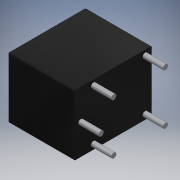
# Autodesk Inventor part: VAR-RELAY-12V10A-CHICO
Saved by Autodesk Inventor 2018.3 (Build 223284000, 284)
## iProperties
Created: 2021-05-31
Part Number: VAR-RELAY-12V10A-CHICO
Material: Genérico
Document SubType Name: Modeling
Designer: laguerre
Density: 8.47 g/cm^3
Appearance: Suave - Negro
Author: laguerre
Autodesk Inventor part; units mm, degrees
note: some values were not read from the file. Chosen so that the rebuilt part matches the saved one: direction of "Repujado1".
ref_plane "YZ Plane" through (0, 0, 0) normal (1, 0, 0) x (0, 1, 0)
ref_plane "XZ Plane" through (0, 0, 0) normal (0, 1, 0) x (-1, 0, 0)
ref_plane "XY Plane" through (0, 0, 0) normal (0, 0, 1) x (1, 0, 0)
sketch "Boceto39" plane through (0, 0, 0) normal (0, 0, 1) x (1, 0, 0)
  line L0 (-7.65, 6) -> (7.65, 6)
  line L1 (7.65, 6) -> (7.65, -6)
  line L2 (7.65, -6) -> (-7.65, -6)
  line L3 (-7.65, -6) -> (-7.65, 6)
  point P0 (0, 0)
  point P1 (0, 6)
  point P2 (-7.65, 0)
  dimension "d373" = 15.3
  dimension "d374" = 12
  constraints: 8 end point, 2 midpoint, 2 parallel, 1 horizontal, 1 horizontal alignment, 1 perpendicular, 1 vertical alignment
  measures "d373" distance of L0.start L0.end
  measures "d374" distance of L2.end L0.start
extrude "Extrusión13" add sketch "Boceto39" along normal blind 13.1
sketch "Boceto40" plane through (0, 0, 0) normal (0, 0, -1) x (-1, 0, 0)
  circle A0 centre (-6.35, 0) radius 0.5
  circle A1 centre (-3.85, 5) radius 0.5
  circle A2 centre (-3.85, -5) radius 0.5
  circle A3 centre (6.35, -5) radius 0.5
  circle A4 centre (6.35, 5) radius 0.5
  line L0 (-7.65, 6) -> (-7.65, -6) projected
  point P0 (0, 0)
  dimension "d377" = 2.5
  dimension "d378" = 10.2
  dimension "d379" = 10
  dimension "d380" = 5
  dimension "d381" = 1
  dimension "d382" = 1.3
  constraints: 5 centre point, 4 equal radius, 3 horizontal alignment, 2 vertical alignment
  measures "d377" horizontal distance of A2.centre A0.centre
  measures "d378" distance of A3.centre A2.centre
  measures "d379" distance of A1.centre A2.centre
  measures "d380" vertical distance of A1.centre A0.centre
  measures "d381" diameter of A1
  measures "d382" distance from line of A0.centre L0
extrude "Extrusión14" add sketch "Boceto40" along normal blind 4
fillet "Empalme44" radius 0.2 8 edges at (7.65, 6, 6.55) (7.65, -6, 6.55) (-7.65, 6, 6.55) (-7.65, -6, 6.55) (-7.65, 0, 13.1) (0, -6, 13.1) (7.65, 0, 13.1) (0, 6, 13.1)
sketch "Boceto41" plane through (0, 0, 13.1) normal (0, 0, 1) x (1, 0, 0)
  line L0 (5.3129, 0) -> (-7.1764, 0) construction
  line L1 (-7.1764, 0) -> (-7.1764, 5.3526) construction
  line L2 (-7.1764, 5.3526) -> (5.3129, 5.3526) construction
  line L3 (5.3129, 5.3526) -> (5.3129, 0) construction
  line L4 (4.6233, 1.0211) -> (5.24, 1.0211)
  line L5 (5.24, 1.0211) -> (5.24, 0.8793)
  spline S0 degree 2 poles (5.24, 0.8793) (5.1736, 0.8169) (5.0552, 0.701) (4.9985, 0.6386) knots 0 0 0 1 2 2 2
  spline S1 degree 2 poles (4.9985, 0.6386) (4.8843, 0.513) (4.8008, 0.3622) (4.8008, 0.282) knots 0 0 0 1 2 2 2
  spline S2 degree 2 poles (4.8008, 0.282) (4.8008, 0.2399) (4.8267, 0.1767) (4.8502, 0.1564) knots 0 0 0 1 2 2 2
  spline S3 degree 2 poles (4.8502, 0.1564) (4.8737, 0.1361) (4.9353, 0.1159) (4.9726, 0.1159) knots 0 0 0 1 2 2 2
  spline S4 degree 2 poles (4.9726, 0.1159) (5.0082, 0.1159) (5.0812, 0.1337) (5.1144, 0.1475) knots 0 0 0 1 2 2 2
  spline S5 degree 2 poles (5.1144, 0.1475) (5.1428, 0.1588) (5.1954, 0.1912) (5.2116, 0.2026) knots 0 0 0 1 2 2 2
  line L6 (5.2116, 0.2026) -> (5.2189, 0.2026)
  line L7 (5.2189, 0.2026) -> (5.2189, 0.06)
  spline S6 degree 2 poles (5.2189, 0.06) (5.1776, 0.0397) (5.0293, 0) (4.9629, 0) knots 0 0 0 1 2 2 2
  spline S7 degree 2 poles (4.9629, 0) (4.8227, 0) (4.6646, 0.1483) (4.6646, 0.2747) knots 0 0 0 1 2 2 2
  spline S8 degree 2 poles (4.6646, 0.2747) (4.6646, 0.3339) (4.6922, 0.4327) (4.7165, 0.4749) knots 0 0 0 1 2 2 2
  spline S9 degree 2 poles (4.7165, 0.4749) (4.7408, 0.5186) (4.8113, 0.6045) (4.8502, 0.6459) knots 0 0 0 1 2 2 2
  spline S10 degree 2 poles (4.8502, 0.6459) (4.9134, 0.7147) (5.0682, 0.8622) (5.1144, 0.9052) knots 0 0 0 1 2 2 2
  line L8 (5.1144, 0.9052) -> (4.6233, 0.9052)
  line L9 (4.6233, 0.9052) -> (4.6233, 1.0211)
  spline S11 degree 2 poles (3.8672, 0.5211) (3.8672, 0.7901) (4.0236, 1.0421) (4.1865, 1.0421) knots 0 0 0 1 2 2 2
  spline S12 degree 2 poles (4.1865, 1.0421) (4.3518, 1.0421) (4.5066, 0.7853) (4.5066, 0.5219) knots 0 0 0 1 2 2 2
  spline S13 degree 2 poles (4.5066, 0.5219) (4.5066, 0.2512) (4.3502, 0.0008) (4.1865, 0.0008) knots 0 0 0 1 2 2 2
  spline S14 degree 2 poles (4.1865, 0.0008) (4.022, 0.0008) (3.8672, 0.2601) (3.8672, 0.5211) knots 0 0 0 1 2 2 2
  spline S15 degree 2 poles (4.039, 0.8258) (4.0196, 0.7763) (4.0034, 0.624) (4.0034, 0.5211) knots 0 0 0 1 2 2 2
  spline S16 degree 2 poles (4.0034, 0.5211) (4.0034, 0.4182) (4.0196, 0.2666) (4.0398, 0.2156) knots 0 0 0 1 2 2 2
  spline S17 degree 2 poles (4.0398, 0.2156) (4.0601, 0.1645) (4.1306, 0.1118) (4.1865, 0.1118) knots 0 0 0 1 2 2 2
  spline S18 degree 2 poles (4.1865, 0.1118) (4.2424, 0.1118) (4.3146, 0.1645) (4.3356, 0.2172) knots 0 0 0 1 2 2 2
  spline S19 degree 2 poles (4.3356, 0.2172) (4.3559, 0.2682) (4.3705, 0.4238) (4.3705, 0.5219) knots 0 0 0 1 2 2 2
  spline S20 degree 2 poles (4.3705, 0.5219) (4.3705, 0.6272) (4.3575, 0.7682) (4.3364, 0.8233) knots 0 0 0 1 2 2 2
  spline S21 degree 2 poles (4.3364, 0.8233) (4.317, 0.8752) (4.2449, 0.9311) (4.1865, 0.9311) knots 0 0 0 1 2 2 2
  spline S22 degree 2 poles (4.1865, 0.9311) (4.1314, 0.9311) (4.0593, 0.8784) (4.039, 0.8258) knots 0 0 0 1 2 2 2
  line L10 (3.8186, 1.0211) -> (3.4815, 0.0211)
  line L11 (3.4815, 0.0211) -> (3.3178, 0.0211)
  line L12 (3.3178, 0.0211) -> (2.9807, 1.0211)
  line L13 (2.9807, 1.0211) -> (3.1209, 1.0211)
  line L14 (3.1209, 1.0211) -> (3.2116, 0.7415)
  line L15 (3.2116, 0.7415) -> (3.5933, 0.7415)
  line L16 (3.5933, 0.7415) -> (3.6841, 1.0211)
  line L17 (3.6841, 1.0211) -> (3.8186, 1.0211)
  line L18 (3.2481, 0.628) -> (3.4029, 0.1572)
  line L19 (3.4029, 0.1572) -> (3.5569, 0.628)
  line L20 (3.5569, 0.628) -> (3.2481, 0.628)
  line L21 (0.2003, 1.0211) -> (0.6881, 1.0211)
  line L22 (0.6881, 1.0211) -> (0.6881, 0.919)
  line L23 (0.6881, 0.919) -> (0.5066, 0.919)
  line L24 (0.5066, 0.919) -> (0.5066, 0.2488)
  line L25 (0.5066, 0.2488) -> (0.6881, 0.2488)
  line L26 (0.6881, 0.2488) -> (0.6881, 0.1572)
  spline S23 degree 2 poles (0.6881, 0.1572) (0.5852, 0.1572) (0.488, 0.0989) (0.4815, 0.0178) knots 0 0 0 1 2 2 2
  line L27 (0.4815, 0.0178) -> (0.3778, 0.0178)
  line L28 (0.3778, 0.0178) -> (0.3778, 0.919)
  line L29 (0.3778, 0.919) -> (0.2003, 0.919)
  line L30 (0.2003, 0.919) -> (0.2003, 1.0211)
  line L31 (-0.6004, 1.0211) -> (0.0163, 1.0211)
  line L32 (0.0163, 1.0211) -> (0.0163, 0.8793)
  spline S24 degree 2 poles (0.0163, 0.8793) (-0.0501, 0.8169) (-0.1684, 0.701) (-0.2251, 0.6386) knots 0 0 0 1 2 2 2
  spline S25 degree 2 poles (-0.2251, 0.6386) (-0.3394, 0.513) (-0.4229, 0.3622) (-0.4229, 0.282) knots 0 0 0 1 2 2 2
  spline S26 degree 2 poles (-0.4229, 0.282) (-0.4229, 0.2399) (-0.3969, 0.1767) (-0.3734, 0.1564) knots 0 0 0 1 2 2 2
  spline S27 degree 2 poles (-0.3734, 0.1564) (-0.3499, 0.1361) (-0.2884, 0.1159) (-0.2511, 0.1159) knots 0 0 0 1 2 2 2
  spline S28 degree 2 poles (-0.2511, 0.1159) (-0.2154, 0.1159) (-0.1425, 0.1337) (-0.1093, 0.1475) knots 0 0 0 1 2 2 2
  spline S29 degree 2 poles (-0.1093, 0.1475) (-0.0809, 0.1588) (-0.0282, 0.1912) (-0.012, 0.2026) knots 0 0 0 1 2 2 2
  line L33 (-0.012, 0.2026) -> (-0.0047, 0.2026)
  line L34 (-0.0047, 0.2026) -> (-0.0047, 0.06)
  spline S30 degree 2 poles (-0.0047, 0.06) (-0.0461, 0.0397) (-0.1944, 0) (-0.2608, 0) knots 0 0 0 1 2 2 2
  spline S31 degree 2 poles (-0.2608, 0) (-0.401, 0) (-0.559, 0.1483) (-0.559, 0.2747) knots 0 0 0 1 2 2 2
  spline S32 degree 2 poles (-0.559, 0.2747) (-0.559, 0.3339) (-0.5315, 0.4327) (-0.5072, 0.4749) knots 0 0 0 1 2 2 2
  spline S33 degree 2 poles (-0.5072, 0.4749) (-0.4828, 0.5186) (-0.4123, 0.6045) (-0.3734, 0.6459) knots 0 0 0 1 2 2 2
  spline S34 degree 2 poles (-0.3734, 0.6459) (-0.3102, 0.7147) (-0.1555, 0.8622) (-0.1093, 0.9052) knots 0 0 0 1 2 2 2
  line L35 (-0.1093, 0.9052) -> (-0.6004, 0.9052)
  line L36 (-0.6004, 0.9052) -> (-0.6004, 1.0211)
  spline S35 degree 2 poles (-1.3402, 0.7034) (-1.3402, 0.7755) (-1.294, 0.8987) (-1.2519, 0.9441) knots 0 0 0 1 2 2 2
  spline S36 degree 2 poles (-1.2519, 0.9441) (-1.2098, 0.9895) (-1.0841, 1.0421) (-1.0063, 1.0421) knots 0 0 0 1 2 2 2
  spline S37 degree 2 poles (-1.0063, 1.0421) (-0.935, 1.0421) (-0.7957, 1.0105) (-0.7446, 0.9854) knots 0 0 0 1 2 2 2
  line L37 (-0.7446, 0.9854) -> (-0.7446, 0.8436)
  line L38 (-0.7446, 0.8436) -> (-0.7543, 0.8436)
  spline S38 degree 2 poles (-0.7543, 0.8436) (-0.7697, 0.8549) (-0.8273, 0.8841) (-0.8621, 0.8971) knots 0 0 0 1 2 2 2
  spline S39 degree 2 poles (-0.8621, 0.8971) (-0.9018, 0.9109) (-0.9674, 0.9263) (-1.0088, 0.9263) knots 0 0 0 1 2 2 2
  spline S40 degree 2 poles (-1.0088, 0.9263) (-1.0493, 0.9263) (-1.1255, 0.8971) (-1.153, 0.8655) knots 0 0 0 1 2 2 2
  spline S41 degree 2 poles (-1.153, 0.8655) (-1.1781, 0.8355) (-1.2041, 0.7561) (-1.2041, 0.7026) knots 0 0 0 1 2 2 2
  spline S42 degree 2 poles (-1.2041, 0.7026) (-1.2041, 0.6491) (-1.1749, 0.581) (-1.1474, 0.5583) knots 0 0 0 1 2 2 2
  spline S43 degree 2 poles (-1.1474, 0.5583) (-1.119, 0.5332) (-1.0347, 0.5122) (-0.9837, 0.5122) knots 0 0 0 1 2 2 2
  spline S44 degree 2 poles (-0.9837, 0.5122) (-0.9286, 0.5122) (-0.8192, 0.5292) (-0.7859, 0.5365) knots 0 0 0 1 2 2 2
  line L39 (-0.7859, 0.5365) -> (-0.7859, 0.0211)
  line L40 (-0.7859, 0.0211) -> (-1.3345, 0.0211)
  line L41 (-1.3345, 0.0211) -> (-1.3345, 0.1386)
  line L42 (-1.3345, 0.1386) -> (-0.9148, 0.1386)
  line L43 (-0.9148, 0.1386) -> (-0.9148, 0.4052)
  spline S45 degree 2 poles (-0.9148, 0.4052) (-0.9391, 0.4019) (-0.9861, 0.3995) (-1.0055, 0.3995) knots 0 0 0 1 2 2 2
  spline S46 degree 2 poles (-1.0055, 0.3995) (-1.0825, 0.3995) (-1.1887, 0.4246) (-1.2373, 0.4619) knots 0 0 0 1 2 2 2
  spline S47 degree 2 poles (-1.2373, 0.4619) (-1.2867, 0.4992) (-1.3402, 0.6126) (-1.3402, 0.7034) knots 0 0 0 1 2 2 2
  line L44 (-2.2381, 0.0211) -> (-1.8937, 1.0211)
  line L45 (-1.8937, 1.0211) -> (-1.7503, 1.0211)
  line L46 (-1.7503, 1.0211) -> (-1.4059, 0.0211)
  line L47 (-1.4059, 0.0211) -> (-1.5485, 0.0211)
  line L48 (-1.5485, 0.0211) -> (-1.8256, 0.8517)
  line L49 (-1.8256, 0.8517) -> (-2.1028, 0.0211)
  line L50 (-2.1028, 0.0211) -> (-2.2381, 0.0211)
  line L51 (-2.226, 1.0211) -> (-2.5631, 0.0211)
  line L52 (-2.5631, 0.0211) -> (-2.7268, 0.0211)
  line L53 (-2.7268, 0.0211) -> (-3.0639, 1.0211)
  line L54 (-3.0639, 1.0211) -> (-2.9237, 1.0211)
  line L55 (-2.9237, 1.0211) -> (-2.8329, 0.7415)
  line L56 (-2.8329, 0.7415) -> (-2.4512, 0.7415)
  line L57 (-2.4512, 0.7415) -> (-2.3605, 1.0211)
  line L58 (-2.3605, 1.0211) -> (-2.226, 1.0211)
  line L59 (-2.7965, 0.628) -> (-2.6417, 0.1572)
  line L60 (-2.6417, 0.1572) -> (-2.4877, 0.628)
  line L61 (-2.4877, 0.628) -> (-2.7965, 0.628)
  spline S48 degree 2 poles (-3.5493, 1.0389) (-3.4521, 1.0389) (-3.2875, 0.9733) (-3.2276, 0.9076) knots 0 0 0 1 2 2 2
  spline S49 degree 2 poles (-3.2276, 0.9076) (-3.1676, 0.8428) (-3.102, 0.6483) (-3.102, 0.5219) knots 0 0 0 1 2 2 2
  spline S50 degree 2 poles (-3.102, 0.5219) (-3.102, 0.3963) (-3.166, 0.2099) (-3.2268, 0.141) knots 0 0 0 1 2 2 2
  spline S51 degree 2 poles (-3.2268, 0.141) (-3.2867, 0.0737) (-3.4504, 0.0032) (-3.5517, 0.0032) knots 0 0 0 1 2 2 2
  spline S52 degree 2 poles (-3.5517, 0.0032) (-3.602, 0.0032) (-3.6903, 0.0178) (-3.7276, 0.0292) knots 0 0 0 1 2 2 2
  spline S53 degree 2 poles (-3.7276, 0.0292) (-3.76, 0.0397) (-3.8273, 0.0697) (-3.8605, 0.0875) knots 0 0 0 1 2 2 2
  line L62 (-3.8605, 0.0875) -> (-3.8605, 0.248)
  line L63 (-3.8605, 0.248) -> (-3.8499, 0.248)
  spline S54 degree 2 poles (-3.8499, 0.248) (-3.8321, 0.2318) (-3.777, 0.1864) (-3.7373, 0.1645) knots 0 0 0 1 2 2 2
  spline S55 degree 2 poles (-3.7373, 0.1645) (-3.6992, 0.1434) (-3.6093, 0.1167) (-3.5509, 0.1167) knots 0 0 0 1 2 2 2
  spline S56 degree 2 poles (-3.5509, 0.1167) (-3.4869, 0.1167) (-3.3726, 0.1694) (-3.3297, 0.2196) knots 0 0 0 1 2 2 2
  spline S57 degree 2 poles (-3.3297, 0.2196) (-3.2875, 0.2707) (-3.2405, 0.4254) (-3.2405, 0.5219) knots 0 0 0 1 2 2 2
  spline S58 degree 2 poles (-3.2405, 0.5219) (-3.2405, 0.6248) (-3.29, 0.7731) (-3.3329, 0.8241) knots 0 0 0 1 2 2 2
  spline S59 degree 2 poles (-3.3329, 0.8241) (-3.3751, 0.8736) (-3.4877, 0.9238) (-3.5509, 0.9238) knots 0 0 0 1 2 2 2
  spline S60 degree 2 poles (-3.5509, 0.9238) (-3.6085, 0.9238) (-3.7065, 0.8955) (-3.7446, 0.8744) knots 0 0 0 1 2 2 2
  spline S61 degree 2 poles (-3.7446, 0.8744) (-3.7811, 0.8533) (-3.8354, 0.8096) (-3.8508, 0.7942) knots 0 0 0 1 2 2 2
  line L64 (-3.8508, 0.7942) -> (-3.8605, 0.7942)
  line L65 (-3.8605, 0.7942) -> (-3.8605, 0.953)
  spline S62 degree 2 poles (-3.8605, 0.953) (-3.8273, 0.9684) (-3.7689, 0.9968) (-3.7276, 1.0097) knots 0 0 0 1 2 2 2
  spline S63 degree 2 poles (-3.7276, 1.0097) (-3.6838, 1.0243) (-3.6093, 1.0389) (-3.5493, 1.0389) knots 0 0 0 1 2 2 2
  line L66 (4.6233, 2.6675) -> (5.24, 2.6675)
  line L67 (5.24, 2.6675) -> (5.24, 2.5257)
  spline S64 degree 2 poles (5.24, 2.5257) (5.1736, 2.4633) (5.0552, 2.3474) (4.9985, 2.285) knots 0 0 0 1 2 2 2
  spline S65 degree 2 poles (4.9985, 2.285) (4.8843, 2.1594) (4.8008, 2.0087) (4.8008, 1.9285) knots 0 0 0 1 2 2 2
  spline S66 degree 2 poles (4.8008, 1.9285) (4.8008, 1.8863) (4.8267, 1.8231) (4.8502, 1.8029) knots 0 0 0 1 2 2 2
  spline S67 degree 2 poles (4.8502, 1.8029) (4.8737, 1.7826) (4.9353, 1.7624) (4.9726, 1.7624) knots 0 0 0 1 2 2 2
  spline S68 degree 2 poles (4.9726, 1.7624) (5.0082, 1.7624) (5.0812, 1.7802) (5.1144, 1.794) knots 0 0 0 1 2 2 2
  spline S69 degree 2 poles (5.1144, 1.794) (5.1428, 1.8053) (5.1954, 1.8377) (5.2116, 1.8491) knots 0 0 0 1 2 2 2
  line L68 (5.2116, 1.8491) -> (5.2189, 1.8491)
  line L69 (5.2189, 1.8491) -> (5.2189, 1.7064)
  spline S70 degree 2 poles (5.2189, 1.7064) (5.1776, 1.6862) (5.0293, 1.6465) (4.9629, 1.6465) knots 0 0 0 1 2 2 2
  spline S71 degree 2 poles (4.9629, 1.6465) (4.8227, 1.6465) (4.6646, 1.7948) (4.6646, 1.9212) knots 0 0 0 1 2 2 2
  spline S72 degree 2 poles (4.6646, 1.9212) (4.6646, 1.9803) (4.6922, 2.0792) (4.7165, 2.1214) knots 0 0 0 1 2 2 2
  spline S73 degree 2 poles (4.7165, 2.1214) (4.7408, 2.1651) (4.8113, 2.251) (4.8502, 2.2923) knots 0 0 0 1 2 2 2
  spline S74 degree 2 poles (4.8502, 2.2923) (4.9134, 2.3612) (5.0682, 2.5087) (5.1144, 2.5517) knots 0 0 0 1 2 2 2
  line L70 (5.1144, 2.5517) -> (4.6233, 2.5517)
  line L71 (4.6233, 2.5517) -> (4.6233, 2.6675)
  spline S75 degree 2 poles (3.8672, 2.1675) (3.8672, 2.4366) (4.0236, 2.6886) (4.1865, 2.6886) knots 0 0 0 1 2 2 2
  spline S76 degree 2 poles (4.1865, 2.6886) (4.3518, 2.6886) (4.5066, 2.4317) (4.5066, 2.1684) knots 0 0 0 1 2 2 2
  spline S77 degree 2 poles (4.5066, 2.1684) (4.5066, 1.8977) (4.3502, 1.6473) (4.1865, 1.6473) knots 0 0 0 1 2 2 2
  spline S78 degree 2 poles (4.1865, 1.6473) (4.022, 1.6473) (3.8672, 1.9066) (3.8672, 2.1675) knots 0 0 0 1 2 2 2
  spline S79 degree 2 poles (4.039, 2.4722) (4.0196, 2.4228) (4.0034, 2.2705) (4.0034, 2.1675) knots 0 0 0 1 2 2 2
  spline S80 degree 2 poles (4.0034, 2.1675) (4.0034, 2.0646) (4.0196, 1.9131) (4.0398, 1.862) knots 0 0 0 1 2 2 2
  spline S81 degree 2 poles (4.0398, 1.862) (4.0601, 1.811) (4.1306, 1.7583) (4.1865, 1.7583) knots 0 0 0 1 2 2 2
  spline S82 degree 2 poles (4.1865, 1.7583) (4.2424, 1.7583) (4.3146, 1.811) (4.3356, 1.8637) knots 0 0 0 1 2 2 2
  spline S83 degree 2 poles (4.3356, 1.8637) (4.3559, 1.9147) (4.3705, 2.0703) (4.3705, 2.1684) knots 0 0 0 1 2 2 2
  spline S84 degree 2 poles (4.3705, 2.1684) (4.3705, 2.2737) (4.3575, 2.4147) (4.3364, 2.4698) knots 0 0 0 1 2 2 2
  spline S85 degree 2 poles (4.3364, 2.4698) (4.317, 2.5217) (4.2449, 2.5776) (4.1865, 2.5776) knots 0 0 0 1 2 2 2
  spline S86 degree 2 poles (4.1865, 2.5776) (4.1314, 2.5776) (4.0593, 2.5249) (4.039, 2.4722) knots 0 0 0 1 2 2 2
  line L72 (3.8186, 2.6675) -> (3.4815, 1.6675)
  line L73 (3.4815, 1.6675) -> (3.3178, 1.6675)
  line L74 (3.3178, 1.6675) -> (2.9807, 2.6675)
  line L75 (2.9807, 2.6675) -> (3.1209, 2.6675)
  line L76 (3.1209, 2.6675) -> (3.2116, 2.388)
  line L77 (3.2116, 2.388) -> (3.5933, 2.388)
  line L78 (3.5933, 2.388) -> (3.6841, 2.6675)
  line L79 (3.6841, 2.6675) -> (3.8186, 2.6675)
  line L80 (3.2481, 2.2745) -> (3.4029, 1.8037)
  line L81 (3.4029, 1.8037) -> (3.5569, 2.2745)
  line L82 (3.5569, 2.2745) -> (3.2481, 2.2745)
  line L83 (0.2003, 2.6675) -> (0.6881, 2.6675)
  line L84 (0.6881, 2.6675) -> (0.6881, 2.5654)
  line L85 (0.6881, 2.5654) -> (0.5066, 2.5654)
  line L86 (0.5066, 2.5654) -> (0.5066, 1.8953)
  line L87 (0.5066, 1.8953) -> (0.6881, 1.8953)
  line L88 (0.6881, 1.8953) -> (0.6881, 1.8037)
  spline S87 degree 2 poles (0.6881, 1.8037) (0.5852, 1.8037) (0.488, 1.7453) (0.4815, 1.6643) knots 0 0 0 1 2 2 2
  line L89 (0.4815, 1.6643) -> (0.3778, 1.6643)
  line L90 (0.3778, 1.6643) -> (0.3778, 2.5654)
  line L91 (0.3778, 2.5654) -> (0.2003, 2.5654)
  line L92 (0.2003, 2.5654) -> (0.2003, 2.6675)
  line L93 (-0.6271, 2.3239) -> (-0.508, 2.3239)
  line L94 (-0.508, 2.3239) -> (-0.508, 2.6675)
  line L95 (-0.508, 2.6675) -> (-0.3791, 2.6675)
  line L96 (-0.3791, 2.6675) -> (-0.3791, 2.3239)
  line L97 (-0.3791, 2.3239) -> (0.0625, 2.3239)
  line L98 (0.0625, 2.3239) -> (0.0625, 2.1829)
  line L99 (0.0625, 2.1829) -> (-0.3848, 1.6675)
  line L100 (-0.3848, 1.6675) -> (-0.508, 1.6675)
  line L101 (-0.508, 1.6675) -> (-0.508, 2.2162)
  line L102 (-0.508, 2.2162) -> (-0.6271, 2.2162)
  line L103 (-0.6271, 2.2162) -> (-0.6271, 2.3239)
  line L104 (-0.3791, 2.2162) -> (-0.3791, 1.8256)
  line L105 (-0.3791, 1.8256) -> (-0.0428, 2.2162)
  line L106 (-0.0428, 2.2162) -> (-0.3791, 2.2162)
  line L107 (-1.4877, 1.6675) -> (-1.1433, 2.6675)
  line L108 (-1.1433, 2.6675) -> (-0.9999, 2.6675)
  line L109 (-0.9999, 2.6675) -> (-0.6555, 1.6675)
  line L110 (-0.6555, 1.6675) -> (-0.7981, 1.6675)
  line L111 (-0.7981, 1.6675) -> (-1.0752, 2.4982)
  line L112 (-1.0752, 2.4982) -> (-1.3524, 1.6675)
  line L113 (-1.3524, 1.6675) -> (-1.4877, 1.6675)
  spline S88 degree 2 poles (-2.3718, 2.1684) (-2.3718, 2.3053) (-2.2608, 2.5257) (-2.1676, 2.5873) knots 0 0 0 1 2 2 2
  spline S89 degree 2 poles (-2.1676, 2.5873) (-2.0914, 2.6351) (-1.935, 2.6675) (-1.8135, 2.6675) knots 0 0 0 1 2 2 2
  line L114 (-1.8135, 2.6675) -> (-1.5833, 2.6675)
  line L115 (-1.5833, 2.6675) -> (-1.5833, 1.6675)
  line L116 (-1.5833, 1.6675) -> (-1.811, 1.6675)
  spline S90 degree 2 poles (-1.811, 1.6675) (-1.9521, 1.6675) (-2.1125, 1.7097) (-2.1692, 1.747) knots 0 0 0 1 2 2 2
  spline S91 degree 2 poles (-2.1692, 1.747) (-2.2657, 1.811) (-2.3718, 2.0225) (-2.3718, 2.1684) knots 0 0 0 1 2 2 2
  spline S92 degree 2 poles (-2.2333, 2.1667) (-2.2333, 2.0517) (-2.1571, 1.8888) (-2.0817, 1.8426) knots 0 0 0 1 2 2 2
  spline S93 degree 2 poles (-2.0817, 1.8426) (-2.0282, 1.811) (-1.9075, 1.7826) (-1.8175, 1.7826) knots 0 0 0 1 2 2 2
  line L117 (-1.8175, 1.7826) -> (-1.7162, 1.7826)
  line L118 (-1.7162, 1.7826) -> (-1.7162, 2.5525)
  line L119 (-1.7162, 2.5525) -> (-1.8175, 2.5525)
  spline S94 degree 2 poles (-1.8175, 2.5525) (-1.9059, 2.5525) (-2.0396, 2.5241) (-2.0939, 2.486) knots 0 0 0 1 2 2 2
  spline S95 degree 2 poles (-2.0939, 2.486) (-2.1636, 2.439) (-2.2333, 2.2834) (-2.2333, 2.1667) knots 0 0 0 1 2 2 2
  spline S96 degree 2 poles (-2.9067, 2.6854) (-2.8094, 2.6854) (-2.6449, 2.6197) (-2.585, 2.5541) knots 0 0 0 1 2 2 2
  spline S97 degree 2 poles (-2.585, 2.5541) (-2.525, 2.4893) (-2.4593, 2.2948) (-2.4593, 2.1684) knots 0 0 0 1 2 2 2
  spline S98 degree 2 poles (-2.4593, 2.1684) (-2.4593, 2.0427) (-2.5234, 1.8564) (-2.5841, 1.7875) knots 0 0 0 1 2 2 2
  spline S99 degree 2 poles (-2.5841, 1.7875) (-2.6441, 1.7202) (-2.8078, 1.6497) (-2.9091, 1.6497) knots 0 0 0 1 2 2 2
  spline S100 degree 2 poles (-2.9091, 1.6497) (-2.9593, 1.6497) (-3.0477, 1.6643) (-3.085, 1.6756) knots 0 0 0 1 2 2 2
  spline S101 degree 2 poles (-3.085, 1.6756) (-3.1174, 1.6862) (-3.1846, 1.7162) (-3.2179, 1.734) knots 0 0 0 1 2 2 2
  line L120 (-3.2179, 1.734) -> (-3.2179, 1.8944)
  line L121 (-3.2179, 1.8944) -> (-3.2073, 1.8944)
  spline S102 degree 2 poles (-3.2073, 1.8944) (-3.1895, 1.8782) (-3.1344, 1.8329) (-3.0947, 1.811) knots 0 0 0 1 2 2 2
  spline S103 degree 2 poles (-3.0947, 1.811) (-3.0566, 1.7899) (-2.9666, 1.7632) (-2.9083, 1.7632) knots 0 0 0 1 2 2 2
  spline S104 degree 2 poles (-2.9083, 1.7632) (-2.8443, 1.7632) (-2.73, 1.8158) (-2.6871, 1.8661) knots 0 0 0 1 2 2 2
  spline S105 degree 2 poles (-2.6871, 1.8661) (-2.6449, 1.9171) (-2.5979, 2.0719) (-2.5979, 2.1684) knots 0 0 0 1 2 2 2
  spline S106 degree 2 poles (-2.5979, 2.1684) (-2.5979, 2.2713) (-2.6474, 2.4196) (-2.6903, 2.4706) knots 0 0 0 1 2 2 2
  spline S107 degree 2 poles (-2.6903, 2.4706) (-2.7324, 2.5201) (-2.8451, 2.5703) (-2.9083, 2.5703) knots 0 0 0 1 2 2 2
  spline S108 degree 2 poles (-2.9083, 2.5703) (-2.9658, 2.5703) (-3.0639, 2.5419) (-3.102, 2.5209) knots 0 0 0 1 2 2 2
  spline S109 degree 2 poles (-3.102, 2.5209) (-3.1384, 2.4998) (-3.1927, 2.456) (-3.2081, 2.4406) knots 0 0 0 1 2 2 2
  line L122 (-3.2081, 2.4406) -> (-3.2179, 2.4406)
  line L123 (-3.2179, 2.4406) -> (-3.2179, 2.5995)
  spline S110 degree 2 poles (-3.2179, 2.5995) (-3.1846, 2.6149) (-3.1263, 2.6432) (-3.085, 2.6562) knots 0 0 0 1 2 2 2
  spline S111 degree 2 poles (-3.085, 2.6562) (-3.0412, 2.6708) (-2.9666, 2.6854) (-2.9067, 2.6854) knots 0 0 0 1 2 2 2
  line L124 (4.8632, 4.314) -> (5.2505, 4.314)
  line L125 (5.2505, 4.314) -> (5.2505, 4.2119)
  line L126 (5.2505, 4.2119) -> (5.1233, 4.2119)
  line L127 (5.1233, 4.2119) -> (5.1233, 3.4161)
  line L128 (5.1233, 3.4161) -> (5.2505, 3.4161)
  line L129 (5.2505, 3.4161) -> (5.2505, 3.314)
  line L130 (5.2505, 3.314) -> (4.8632, 3.314)
  line L131 (4.8632, 3.314) -> (4.8632, 3.4161)
  line L132 (4.8632, 3.4161) -> (4.9904, 3.4161)
  line L133 (4.9904, 3.4161) -> (4.9904, 4.2119)
  line L134 (4.9904, 4.2119) -> (4.8632, 4.2119)
  line L135 (4.8632, 4.2119) -> (4.8632, 4.314)
  spline S112 degree 2 poles (4.3081, 4.3318) (4.4053, 4.3318) (4.5698, 4.2662) (4.6298, 4.2006) knots 0 0 0 1 2 2 2
  spline S113 degree 2 poles (4.6298, 4.2006) (4.6898, 4.1357) (4.7554, 3.9412) (4.7554, 3.8148) knots 0 0 0 1 2 2 2
  spline S114 degree 2 poles (4.7554, 3.8148) (4.7554, 3.6892) (4.6914, 3.5028) (4.6306, 3.434) knots 0 0 0 1 2 2 2
  spline S115 degree 2 poles (4.6306, 3.434) (4.5706, 3.3667) (4.4069, 3.2962) (4.3056, 3.2962) knots 0 0 0 1 2 2 2
  spline S116 degree 2 poles (4.3056, 3.2962) (4.2554, 3.2962) (4.1671, 3.3108) (4.1298, 3.3221) knots 0 0 0 1 2 2 2
  spline S117 degree 2 poles (4.1298, 3.3221) (4.0974, 3.3327) (4.0301, 3.3626) (3.9969, 3.3805) knots 0 0 0 1 2 2 2
  line L136 (3.9969, 3.3805) -> (3.9969, 3.5409)
  line L137 (3.9969, 3.5409) -> (4.0074, 3.5409)
  spline S118 degree 2 poles (4.0074, 3.5409) (4.0253, 3.5247) (4.0804, 3.4793) (4.1201, 3.4575) knots 0 0 0 1 2 2 2
  spline S119 degree 2 poles (4.1201, 3.4575) (4.1582, 3.4364) (4.2481, 3.4096) (4.3065, 3.4096) knots 0 0 0 1 2 2 2
  spline S120 degree 2 poles (4.3065, 3.4096) (4.3705, 3.4096) (4.4847, 3.4623) (4.5277, 3.5126) knots 0 0 0 1 2 2 2
  spline S121 degree 2 poles (4.5277, 3.5126) (4.5698, 3.5636) (4.6168, 3.7184) (4.6168, 3.8148) knots 0 0 0 1 2 2 2
  spline S122 degree 2 poles (4.6168, 3.8148) (4.6168, 3.9177) (4.5674, 4.066) (4.5244, 4.1171) knots 0 0 0 1 2 2 2
  spline S123 degree 2 poles (4.5244, 4.1171) (4.4823, 4.1665) (4.3697, 4.2168) (4.3065, 4.2168) knots 0 0 0 1 2 2 2
  spline S124 degree 2 poles (4.3065, 4.2168) (4.2489, 4.2168) (4.1509, 4.1884) (4.1128, 4.1673) knots 0 0 0 1 2 2 2
  spline S125 degree 2 poles (4.1128, 4.1673) (4.0763, 4.1463) (4.022, 4.1025) (4.0066, 4.0871) knots 0 0 0 1 2 2 2
  line L138 (4.0066, 4.0871) -> (3.9969, 4.0871)
  line L139 (3.9969, 4.0871) -> (3.9969, 4.2459)
  spline S126 degree 2 poles (3.9969, 4.2459) (4.0301, 4.2613) (4.0885, 4.2897) (4.1298, 4.3027) knots 0 0 0 1 2 2 2
  spline S127 degree 2 poles (4.1298, 4.3027) (4.1736, 4.3173) (4.2481, 4.3318) (4.3081, 4.3318) knots 0 0 0 1 2 2 2
  spline S128 degree 2 poles (3.0423, 4.5587) (3.0787, 4.5677) (3.1582, 4.5774) (3.1979, 4.5774) knots 0 0 0 1 2 2 2
  spline S129 degree 2 poles (3.1979, 4.5774) (3.3105, 4.5774) (3.4507, 4.4518) (3.4572, 4.3351) knots 0 0 0 1 2 2 2
  spline S130 degree 2 poles (3.4572, 4.3351) (3.4661, 4.3351) (3.4815, 4.3351) (3.488, 4.3351) knots 0 0 0 1 2 2 2
  spline S131 degree 2 poles (3.488, 4.3351) (3.5893, 4.3351) (3.7522, 4.2662) (3.8105, 4.1989) knots 0 0 0 1 2 2 2
  spline S132 degree 2 poles (3.8105, 4.1989) (3.868, 4.1325) (3.9296, 3.938) (3.9296, 3.8148) knots 0 0 0 1 2 2 2
  spline S133 degree 2 poles (3.9296, 3.8148) (3.9296, 3.6884) (3.8672, 3.4972) (3.8097, 3.4291) knots 0 0 0 1 2 2 2
  spline S134 degree 2 poles (3.8097, 3.4291) (3.7514, 3.3618) (3.5885, 3.2929) (3.488, 3.2929) knots 0 0 0 1 2 2 2
  spline S135 degree 2 poles (3.488, 3.2929) (3.3859, 3.2929) (3.2222, 3.3643) (3.1655, 3.4291) knots 0 0 0 1 2 2 2
  spline S136 degree 2 poles (3.1655, 3.4291) (3.1087, 3.4947) (3.0455, 3.69) (3.0455, 3.8148) knots 0 0 0 1 2 2 2
  spline S137 degree 2 poles (3.0455, 3.8148) (3.0455, 4.0093) (3.1971, 4.2622) (3.3291, 4.3067) knots 0 0 0 1 2 2 2
  spline S138 degree 2 poles (3.3291, 4.3067) (3.3259, 4.344) (3.3065, 4.404) (3.2911, 4.421) knots 0 0 0 1 2 2 2
  spline S139 degree 2 poles (3.2911, 4.421) (3.2724, 4.4421) (3.2214, 4.4615) (3.176, 4.4615) knots 0 0 0 1 2 2 2
  spline S140 degree 2 poles (3.176, 4.4615) (3.1492, 4.4615) (3.0763, 4.4445) (3.0601, 4.438) knots 0 0 0 1 2 2 2
  line L140 (3.0601, 4.438) -> (3.0423, 4.438)
  line L141 (3.0423, 4.438) -> (3.0423, 4.5587)
  spline S141 degree 2 poles (3.1841, 3.8148) (3.1841, 3.7152) (3.227, 3.562) (3.2659, 3.5117) knots 0 0 0 1 2 2 2
  spline S142 degree 2 poles (3.2659, 3.5117) (3.3056, 3.4599) (3.4175, 3.408) (3.4872, 3.408) knots 0 0 0 1 2 2 2
  spline S143 degree 2 poles (3.4872, 3.408) (3.5593, 3.408) (3.6679, 3.4583) (3.7092, 3.5117) knots 0 0 0 1 2 2 2
  spline S144 degree 2 poles (3.7092, 3.5117) (3.7489, 3.5628) (3.7911, 3.7176) (3.7911, 3.8148) knots 0 0 0 1 2 2 2
  spline S145 degree 2 poles (3.7911, 3.8148) (3.7911, 4.0117) (3.6257, 4.2216) (3.4872, 4.2216) knots 0 0 0 1 2 2 2
  spline S146 degree 2 poles (3.4872, 4.2216) (3.3486, 4.2216) (3.1841, 4.0117) (3.1841, 3.8148) knots 0 0 0 1 2 2 2
  line L142 (2.5617, 3.9372) -> (2.9402, 3.9372)
  line L143 (2.9402, 3.9372) -> (2.9402, 3.8156)
  line L144 (2.9402, 3.8156) -> (2.5617, 3.8156)
  line L145 (2.5617, 3.8156) -> (2.5617, 3.9372)
  line L146 (2.1671, 4.314) -> (2.1671, 3.4323)
  line L147 (2.1671, 3.4323) -> (2.5026, 3.4323)
  line L148 (2.5026, 3.4323) -> (2.5026, 3.314)
  line L149 (2.5026, 3.314) -> (1.6987, 3.314)
  line L150 (1.6987, 3.314) -> (1.6987, 3.4323)
  line L151 (1.6987, 3.4323) -> (2.0342, 3.4323)
  line L152 (2.0342, 3.4323) -> (2.0342, 4.314)
  line L153 (2.0342, 4.314) -> (2.1671, 4.314)
  line L154 (0.9977, 3.4639) -> (1.4304, 4.314)
  line L155 (1.4304, 4.314) -> (1.5731, 4.314)
  line L156 (1.5731, 4.314) -> (1.116, 3.4315)
  line L157 (1.116, 3.4315) -> (1.6322, 3.4315)
  line L158 (1.6322, 3.4315) -> (1.6322, 3.314)
  line L159 (1.6322, 3.314) -> (0.9977, 3.314)
  line L160 (0.9977, 3.314) -> (0.9977, 3.4639)
  spline S147 degree 2 poles (0.5731, 4.3367) (0.6476, 4.3367) (0.77, 4.2921) (0.8129, 4.2508) knots 0 0 0 1 2 2 2
  spline S148 degree 2 poles (0.8129, 4.2508) (0.8551, 4.2103) (0.8988, 4.1001) (0.8988, 4.0377) knots 0 0 0 1 2 2 2
  spline S149 degree 2 poles (0.8988, 4.0377) (0.8988, 3.9566) (0.8121, 3.8205) (0.7295, 3.78) knots 0 0 0 1 2 2 2
  line L161 (0.7295, 3.78) -> (0.7295, 3.7759)
  spline S150 degree 2 poles (0.7295, 3.7759) (0.8032, 3.733) (0.8745, 3.6309) (0.8745, 3.5547) knots 0 0 0 1 2 2 2
  spline S151 degree 2 poles (0.8745, 3.5547) (0.8745, 3.4421) (0.7043, 3.2913) (0.5731, 3.2913) knots 0 0 0 1 2 2 2
  spline S152 degree 2 poles (0.5731, 3.2913) (0.4369, 3.2913) (0.2724, 3.434) (0.2724, 3.5458) knots 0 0 0 1 2 2 2
  spline S153 degree 2 poles (0.2724, 3.5458) (0.2724, 3.613) (0.351, 3.7443) (0.4248, 3.7816) knots 0 0 0 1 2 2 2
  line L162 (0.4248, 3.7816) -> (0.4248, 3.7857)
  spline S154 degree 2 poles (0.4248, 3.7857) (0.3373, 3.8262) (0.2473, 3.9429) (0.2473, 4.0352) knots 0 0 0 1 2 2 2
  spline S155 degree 2 poles (0.2473, 4.0352) (0.2473, 4.1633) (0.4337, 4.3367) (0.5731, 4.3367) knots 0 0 0 1 2 2 2
  spline S156 degree 2 poles (0.3851, 4.0482) (0.3851, 3.9866) (0.4337, 3.9137) (0.5026, 3.8764) knots 0 0 0 1 2 2 2
  spline S157 degree 2 poles (0.5026, 3.8764) (0.5253, 3.8634) (0.6014, 3.8335) (0.6492, 3.814) knots 0 0 0 1 2 2 2
  spline S158 degree 2 poles (0.6492, 3.814) (0.7043, 3.8505) (0.7635, 3.9591) (0.7635, 4.028) knots 0 0 0 1 2 2 2
  spline S159 degree 2 poles (0.7635, 4.028) (0.7635, 4.1187) (0.6541, 4.237) (0.5714, 4.237) knots 0 0 0 1 2 2 2
  spline S160 degree 2 poles (0.5714, 4.237) (0.4872, 4.237) (0.3851, 4.1357) (0.3851, 4.0482) knots 0 0 0 1 2 2 2
  spline S161 degree 2 poles (0.4037, 3.5474) (0.4037, 3.4801) (0.4937, 3.3902) (0.5739, 3.3902) knots 0 0 0 1 2 2 2
  spline S162 degree 2 poles (0.5739, 3.3902) (0.6468, 3.3902) (0.74, 3.4704) (0.74, 3.5393) knots 0 0 0 1 2 2 2
  spline S163 degree 2 poles (0.74, 3.5393) (0.74, 3.5887) (0.6922, 3.6576) (0.6444, 3.6852) knots 0 0 0 1 2 2 2
  spline S164 degree 2 poles (0.6444, 3.6852) (0.6241, 3.6965) (0.5382, 3.7362) (0.5034, 3.7476) knots 0 0 0 1 2 2 2
  spline S165 degree 2 poles (0.5034, 3.7476) (0.445, 3.703) (0.4037, 3.6082) (0.4037, 3.5474) knots 0 0 0 1 2 2 2
  line L163 (-0.2414, 3.9372) -> (0.1371, 3.9372)
  line L164 (0.1371, 3.9372) -> (0.1371, 3.8156)
  line L165 (0.1371, 3.8156) -> (-0.2414, 3.8156)
  line L166 (-0.2414, 3.8156) -> (-0.2414, 3.9372)
  spline S166 degree 2 poles (-1.1911, 3.8148) (-1.1911, 3.9518) (-1.0801, 4.1722) (-0.9869, 4.2338) knots 0 0 0 1 2 2 2
  spline S167 degree 2 poles (-0.9869, 4.2338) (-0.9107, 4.2816) (-0.7543, 4.314) (-0.6328, 4.314) knots 0 0 0 1 2 2 2
  line L167 (-0.6328, 4.314) -> (-0.4026, 4.314)
  line L168 (-0.4026, 4.314) -> (-0.4026, 3.314)
  line L169 (-0.4026, 3.314) -> (-0.6303, 3.314)
  spline S168 degree 2 poles (-0.6303, 3.314) (-0.7713, 3.314) (-0.9318, 3.3562) (-0.9885, 3.3934) knots 0 0 0 1 2 2 2
  spline S169 degree 2 poles (-0.9885, 3.3934) (-1.085, 3.4575) (-1.1911, 3.669) (-1.1911, 3.8148) knots 0 0 0 1 2 2 2
  spline S170 degree 2 poles (-1.0525, 3.8132) (-1.0525, 3.6981) (-0.9764, 3.5352) (-0.901, 3.4891) knots 0 0 0 1 2 2 2
  spline S171 degree 2 poles (-0.901, 3.4891) (-0.8475, 3.4575) (-0.7268, 3.4291) (-0.6368, 3.4291) knots 0 0 0 1 2 2 2
  line L170 (-0.6368, 3.4291) -> (-0.5355, 3.4291)
  line L171 (-0.5355, 3.4291) -> (-0.5355, 4.1989)
  line L172 (-0.5355, 4.1989) -> (-0.6368, 4.1989)
  spline S172 degree 2 poles (-0.6368, 4.1989) (-0.7251, 4.1989) (-0.8589, 4.1706) (-0.9132, 4.1325) knots 0 0 0 1 2 2 2
  spline S173 degree 2 poles (-0.9132, 4.1325) (-0.9828, 4.0855) (-1.0525, 3.9299) (-1.0525, 3.8132) knots 0 0 0 1 2 2 2
  spline S174 degree 2 poles (-1.726, 4.3318) (-1.6287, 4.3318) (-1.4642, 4.2662) (-1.4042, 4.2006) knots 0 0 0 1 2 2 2
  spline S175 degree 2 poles (-1.4042, 4.2006) (-1.3443, 4.1357) (-1.2786, 3.9412) (-1.2786, 3.8148) knots 0 0 0 1 2 2 2
  spline S176 degree 2 poles (-1.2786, 3.8148) (-1.2786, 3.6892) (-1.3427, 3.5028) (-1.4034, 3.434) knots 0 0 0 1 2 2 2
  spline S177 degree 2 poles (-1.4034, 3.434) (-1.4634, 3.3667) (-1.6271, 3.2962) (-1.7284, 3.2962) knots 0 0 0 1 2 2 2
  spline S178 degree 2 poles (-1.7284, 3.2962) (-1.7786, 3.2962) (-1.867, 3.3108) (-1.9042, 3.3221) knots 0 0 0 1 2 2 2
  spline S179 degree 2 poles (-1.9042, 3.3221) (-1.9367, 3.3327) (-2.0039, 3.3626) (-2.0371, 3.3805) knots 0 0 0 1 2 2 2
  line L173 (-2.0371, 3.3805) -> (-2.0371, 3.5409)
  line L174 (-2.0371, 3.5409) -> (-2.0266, 3.5409)
  spline S180 degree 2 poles (-2.0266, 3.5409) (-2.0088, 3.5247) (-1.9537, 3.4793) (-1.914, 3.4575) knots 0 0 0 1 2 2 2
  spline S181 degree 2 poles (-1.914, 3.4575) (-1.8759, 3.4364) (-1.7859, 3.4096) (-1.7276, 3.4096) knots 0 0 0 1 2 2 2
  spline S182 degree 2 poles (-1.7276, 3.4096) (-1.6636, 3.4096) (-1.5493, 3.4623) (-1.5063, 3.5126) knots 0 0 0 1 2 2 2
  spline S183 degree 2 poles (-1.5063, 3.5126) (-1.4642, 3.5636) (-1.4172, 3.7184) (-1.4172, 3.8148) knots 0 0 0 1 2 2 2
  spline S184 degree 2 poles (-1.4172, 3.8148) (-1.4172, 3.9177) (-1.4666, 4.066) (-1.5096, 4.1171) knots 0 0 0 1 2 2 2
  spline S185 degree 2 poles (-1.5096, 4.1171) (-1.5517, 4.1665) (-1.6644, 4.2168) (-1.7276, 4.2168) knots 0 0 0 1 2 2 2
  spline S186 degree 2 poles (-1.7276, 4.2168) (-1.7851, 4.2168) (-1.8832, 4.1884) (-1.9213, 4.1673) knots 0 0 0 1 2 2 2
  spline S187 degree 2 poles (-1.9213, 4.1673) (-1.9577, 4.1463) (-2.012, 4.1025) (-2.0274, 4.0871) knots 0 0 0 1 2 2 2
  line L175 (-2.0274, 4.0871) -> (-2.0371, 4.0871)
  line L176 (-2.0371, 4.0871) -> (-2.0371, 4.2459)
  spline S188 degree 2 poles (-2.0371, 4.2459) (-2.0039, 4.2613) (-1.9456, 4.2897) (-1.9042, 4.3027) knots 0 0 0 1 2 2 2
  spline S189 degree 2 poles (-1.9042, 4.3027) (-1.8605, 4.3173) (-1.7859, 4.3318) (-1.726, 4.3318) knots 0 0 0 1 2 2 2
  line L177 (-2.6992, 4.314) -> (-2.2114, 4.314)
  line L178 (-2.2114, 4.314) -> (-2.2114, 4.2119)
  line L179 (-2.2114, 4.2119) -> (-2.3929, 4.2119)
  line L180 (-2.3929, 4.2119) -> (-2.3929, 3.5417)
  line L181 (-2.3929, 3.5417) -> (-2.2114, 3.5417)
  line L182 (-2.2114, 3.5417) -> (-2.2114, 3.4502)
  spline S190 degree 2 poles (-2.2114, 3.4502) (-2.3143, 3.4502) (-2.4115, 3.3918) (-2.418, 3.3108) knots 0 0 0 1 2 2 2
  line L183 (-2.418, 3.3108) -> (-2.5217, 3.3108)
  line L184 (-2.5217, 3.3108) -> (-2.5217, 4.2119)
  line L185 (-2.5217, 4.2119) -> (-2.6992, 4.2119)
  line L186 (-2.6992, 4.2119) -> (-2.6992, 4.314)
  line L187 (-3.4999, 4.314) -> (-2.8832, 4.314)
  line L188 (-2.8832, 4.314) -> (-2.8832, 4.1722)
  spline S191 degree 2 poles (-2.8832, 4.1722) (-2.9496, 4.1098) (-3.0679, 3.9939) (-3.1247, 3.9315) knots 0 0 0 1 2 2 2
  spline S192 degree 2 poles (-3.1247, 3.9315) (-3.2389, 3.8059) (-3.3224, 3.6552) (-3.3224, 3.575) knots 0 0 0 1 2 2 2
  spline S193 degree 2 poles (-3.3224, 3.575) (-3.3224, 3.5328) (-3.2965, 3.4696) (-3.273, 3.4493) knots 0 0 0 1 2 2 2
  spline S194 degree 2 poles (-3.273, 3.4493) (-3.2495, 3.4291) (-3.1879, 3.4088) (-3.1506, 3.4088) knots 0 0 0 1 2 2 2
  spline S195 degree 2 poles (-3.1506, 3.4088) (-3.1149, 3.4088) (-3.042, 3.4267) (-3.0088, 3.4404) knots 0 0 0 1 2 2 2
  spline S196 degree 2 poles (-3.0088, 3.4404) (-2.9804, 3.4518) (-2.9277, 3.4842) (-2.9115, 3.4955) knots 0 0 0 1 2 2 2
  line L189 (-2.9115, 3.4955) -> (-2.9042, 3.4955)
  line L190 (-2.9042, 3.4955) -> (-2.9042, 3.3529)
  spline S197 degree 2 poles (-2.9042, 3.3529) (-2.9456, 3.3327) (-3.0939, 3.2929) (-3.1603, 3.2929) knots 0 0 0 1 2 2 2
  spline S198 degree 2 poles (-3.1603, 3.2929) (-3.3005, 3.2929) (-3.4585, 3.4412) (-3.4585, 3.5677) knots 0 0 0 1 2 2 2
  spline S199 degree 2 poles (-3.4585, 3.5677) (-3.4585, 3.6268) (-3.431, 3.7257) (-3.4067, 3.7678) knots 0 0 0 1 2 2 2
  spline S200 degree 2 poles (-3.4067, 3.7678) (-3.3824, 3.8116) (-3.3119, 3.8975) (-3.273, 3.9388) knots 0 0 0 1 2 2 2
  spline S201 degree 2 poles (-3.273, 3.9388) (-3.2098, 4.0077) (-3.055, 4.1552) (-3.0088, 4.1981) knots 0 0 0 1 2 2 2
  line L191 (-3.0088, 4.1981) -> (-3.4999, 4.1981)
  line L192 (-3.4999, 4.1981) -> (-3.4999, 4.314)
  line L193 (-4.3872, 3.314) -> (-4.0428, 4.314)
  line L194 (-4.0428, 4.314) -> (-3.8994, 4.314)
  line L195 (-3.8994, 4.314) -> (-3.555, 3.314)
  line L196 (-3.555, 3.314) -> (-3.6976, 3.314)
  line L197 (-3.6976, 3.314) -> (-3.9747, 4.1446)
  line L198 (-3.9747, 4.1446) -> (-4.2519, 3.314)
  line L199 (-4.2519, 3.314) -> (-4.3872, 3.314)
  line L200 (-4.8208, 3.9372) -> (-4.4423, 3.9372)
  line L201 (-4.4423, 3.9372) -> (-4.4423, 3.8156)
  line L202 (-4.4423, 3.8156) -> (-4.8208, 3.8156)
  line L203 (-4.8208, 3.8156) -> (-4.8208, 3.9372)
  spline S202 degree 2 poles (-5.3726, 4.3318) (-5.2754, 4.3318) (-5.1109, 4.2662) (-5.0509, 4.2006) knots 0 0 0 1 2 2 2
  spline S203 degree 2 poles (-5.0509, 4.2006) (-4.991, 4.1357) (-4.9253, 3.9412) (-4.9253, 3.8148) knots 0 0 0 1 2 2 2
  spline S204 degree 2 poles (-4.9253, 3.8148) (-4.9253, 3.6892) (-4.9893, 3.5028) (-5.0501, 3.434) knots 0 0 0 1 2 2 2
  spline S205 degree 2 poles (-5.0501, 3.434) (-5.1101, 3.3667) (-5.2738, 3.2962) (-5.3751, 3.2962) knots 0 0 0 1 2 2 2
  spline S206 degree 2 poles (-5.3751, 3.2962) (-5.4253, 3.2962) (-5.5136, 3.3108) (-5.5509, 3.3221) knots 0 0 0 1 2 2 2
  spline S207 degree 2 poles (-5.5509, 3.3221) (-5.5833, 3.3327) (-5.6506, 3.3626) (-5.6838, 3.3805) knots 0 0 0 1 2 2 2
  line L204 (-5.6838, 3.3805) -> (-5.6838, 3.5409)
  line L205 (-5.6838, 3.5409) -> (-5.6733, 3.5409)
  spline S208 degree 2 poles (-5.6733, 3.5409) (-5.6555, 3.5247) (-5.6004, 3.4793) (-5.5606, 3.4575) knots 0 0 0 1 2 2 2
  spline S209 degree 2 poles (-5.5606, 3.4575) (-5.5226, 3.4364) (-5.4326, 3.4096) (-5.3743, 3.4096) knots 0 0 0 1 2 2 2
  spline S210 degree 2 poles (-5.3743, 3.4096) (-5.3102, 3.4096) (-5.196, 3.4623) (-5.153, 3.5126) knots 0 0 0 1 2 2 2
  spline S211 degree 2 poles (-5.153, 3.5126) (-5.1109, 3.5636) (-5.0639, 3.7184) (-5.0639, 3.8148) knots 0 0 0 1 2 2 2
  spline S212 degree 2 poles (-5.0639, 3.8148) (-5.0639, 3.9177) (-5.1133, 4.066) (-5.1563, 4.1171) knots 0 0 0 1 2 2 2
  spline S213 degree 2 poles (-5.1563, 4.1171) (-5.1984, 4.1665) (-5.311, 4.2168) (-5.3743, 4.2168) knots 0 0 0 1 2 2 2
  spline S214 degree 2 poles (-5.3743, 4.2168) (-5.4318, 4.2168) (-5.5298, 4.1884) (-5.5679, 4.1673) knots 0 0 0 1 2 2 2
  spline S215 degree 2 poles (-5.5679, 4.1673) (-5.6044, 4.1463) (-5.6587, 4.1025) (-5.6741, 4.0871) knots 0 0 0 1 2 2 2
  line L206 (-5.6741, 4.0871) -> (-5.6838, 4.0871)
  line L207 (-5.6838, 4.0871) -> (-5.6838, 4.2459)
  spline S216 degree 2 poles (-5.6838, 4.2459) (-5.6506, 4.2613) (-5.5922, 4.2897) (-5.5509, 4.3027) knots 0 0 0 1 2 2 2
  spline S217 degree 2 poles (-5.5509, 4.3027) (-5.5072, 4.3173) (-5.4326, 4.3318) (-5.3726, 4.3318) knots 0 0 0 1 2 2 2
  point P0 (0, 0)
  constraints: 2 other
emboss "Repujado1" sketch "Boceto41" operation add depth 0.001 direction (0, 0, -1)
